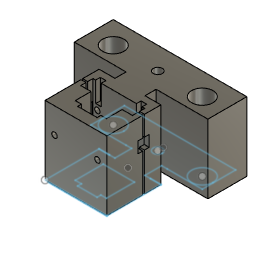
CNC_Assembly (Autodesk Fusion 360 archive; units mm, degrees)
design "spindle handle"
Autodesk Fusion 360 part; units mm, degrees
sketch "Sketch1" plane through (0, 0, 0) normal (0, 0, 1) x (1, 0, 0)
  line L0 (-27.75, -46.75) -> (27.75, -46.75)
  line L1 (27.75, 1.75) -> (27.75, -46.75)
  line L2 (27.75, -46.75) -> (-27.75, -46.75)
  line L3 (14, -8.25) -> (-14, -8.25)
  line L4 (-14, -8.25) -> (-14, -33.35)
  line L5 (-8.5, -36.75) -> (9, -36.75)
  line L6 (14, -33.35) -> (14, -8.25)
  line L7 (-8.5, -36.75) -> (-8.5, -33.35)
  line L8 (-8.5, -33.35) -> (-14, -33.35)
  line L9 (9, -36.75) -> (9, -33.35)
  line L10 (9, -33.35) -> (14, -33.35)
  line L11 (-27.75, 1.75) -> (-18.5, 1.75)
  line L12 (27.75, 1.75) -> (18.5, 1.75)
  circle A0 centre (0, 26.75) radius 4.05
  circle A1 centre (-40, 26.75) radius 9.55
  circle A2 centre (40, 26.75) radius 9.55
  line L13 (50, 46.75) -> (-50, 46.75)
  line L14 (-50, 46.75) -> (-50, 16.75)
  line L15 (50, 16.75) -> (50, 46.75)
  line L16 (-27.75, 1.75) -> (-27.75, -46.75)
  line L17 (-50, 16.75) -> (-18.5, 16.75)
  line L18 (18.5, 16.75) -> (50, 16.75)
  line L19 (-27.75, 1.75) -> (-18.5, 1.75)
  line L20 (18.5, 1.75) -> (27.75, 1.75)
  line L21 (-13.5, 16.75) -> (-13.5, 1.75)
  line L22 (13.5, 1.75) -> (13.5, 16.75)
  line L23 (-18.5, 16.75) -> (-13.5, 16.75)
  line L24 (-18.5, 1.75) -> (-13.5, 1.75)
  line L25 (13.5, 1.75) -> (18.5, 1.75)
  line L26 (13.5, 16.75) -> (18.5, 16.75)
  point P0 (0, 31.75)
  dimension "d19" = 55.5
  dimension "d21" = 48.5
  dimension "d28" = 9.25
  dimension "d29" = 9.25
  dimension "d30" = 15
  dimension "d32" = 8.1
  dimension "d34" = 19.1
  dimension "d36" = 19.1
  dimension "d37" = 100
  dimension "d38" = 30
  dimension "d57" = 27
  dimension "d58" = 15
  dimension "d112" = 28
  dimension "d113" = 17.5
  constraint horizontal L19
  constraint vertical L1
  constraint horizontal L2
  constraint horizontal L3
  constraint perpendicular L3 L4
  constraint parallel L3 L5
  constraint parallel L4 L6
  constraint vertical L7
  constraint horizontal L8
  constraint vertical L9
  constraint horizontal L10
  constraint perpendicular L1 L12
  constraint horizontal L13
  constraint perpendicular L13 L14
  constraint parallel L13 L17
  constraint parallel L14 L15
  constraint collinear L17 L18
  constraint collinear L19 L20
  constraint parallel L21 L22
  constraint perpendicular L21 L23
  measures "d19" distance of L0.start L0.end
  measures "d21" distance of L0.start L11.start
  measures "d28" distance of L11.start L11.end
  measures "d29" distance of L1.start L12.end
  measures "d30" distance of L12.end L18.start
  measures "d32" diameter of A0
  measures "d34" diameter of A1
  measures "d36" diameter of A2
  measures "d37" distance of L14.end L15.start
  measures "d38" distance of L13.end L14.end
  measures "d57" distance of L21.end L22.start
  measures "d58" distance of L21.start L21.end
  measures "d112" distance of L3.start L3.end
  measures "d113" distance of L5.start L5.end
extrude "Extrude4" add sketch "Sketch1" along normal blind 62 makes body 1
sketch "Sketch6" plane through (0, 1.75, 0) normal (0, 1, 0) x (-1, 0, 0)
  line L0 (-27.75, 0) -> (-13.5, 0)
  line L1 (-13.5, 0) -> (-13.5, 62)
  line L2 (-13.5, 62) -> (-27.75, 62)
  line L3 (-27.75, 62) -> (-27.75, 0)
  circle A0 centre (-19.3, 39.2) radius 2.45
  dimension "d63" = 4.9
  measures "d63" diameter of A0
extrude "Extrude5" cut sketch "Sketch6" against normal blind 15 contours A0 bodies 1
sketch "Sketch7" plane through (0, 1.75, 0) normal (0, 1, 0) x (-1, 0, 0)
  line L0 (13.5, 0) -> (27.75, 0)
  line L1 (27.75, 0) -> (27.75, 62)
  line L2 (27.75, 62) -> (13.5, 62)
  line L3 (13.5, 62) -> (13.5, 0)
  circle A0 centre (19.3, 39.2) radius 2.45
  dimension "d71" = 4.9
  measures "d71" diameter of A0
extrude "Extrude6" cut sketch "Sketch7" against normal blind 15 contours A0 bodies 1
sketch "Sketch8" plane through (0, 0, 62) normal (0, 0, 1) x (-1, 0, 0)
  circle A0 centre (0, -26.75) radius 4.05
  circle A1 centre (40, -26.75) radius 9.55
  line L0 (-9, 36.75) -> (8.5, 36.75)
  line L1 (8.5, 36.75) -> (8.5, 33.35)
  line L2 (8.5, 33.35) -> (14, 33.35)
  line L3 (14, 33.35) -> (14, 8.25)
  line L4 (14, 8.25) -> (-14, 8.25)
  line L5 (-14, 8.25) -> (-14, 33.35)
  line L6 (-14, 33.35) -> (-9, 33.35)
  line L7 (-9, 33.35) -> (-9, 36.75)
  circle A2 centre (-40, -26.75) radius 9.55
  line L8 (-13.5, -1.75) -> (-13.5, -16.75)
  line L9 (-13.5, -16.75) -> (-50, -16.75)
  line L10 (-50, -16.75) -> (-50, -46.75)
  line L11 (-50, -46.75) -> (50, -46.75)
  line L12 (50, -46.75) -> (50, -16.75)
  line L13 (50, -16.75) -> (13.5, -16.75)
  line L14 (13.5, -16.75) -> (13.5, -1.75)
  line L15 (13.5, -1.75) -> (27.75, -1.75)
  line L16 (27.75, -1.75) -> (27.75, 46.75)
  line L17 (27.75, 46.75) -> (-27.75, 46.75)
  line L18 (-27.75, 46.75) -> (-27.75, -1.75)
  line L19 (-27.75, -1.75) -> (-13.5, -1.75)
  line L20 (14, 8.25) -> (23.25, 8.25)
  line L21 (23.25, 8.25) -> (23.25, 19.25)
  line L22 (23.25, 19.25) -> (14, 19.25)
  line L23 (14, 19.25) -> (14, 8.25)
  line L24 (-14, 8.25) -> (-23.25, 8.25)
  line L25 (-23.25, 8.25) -> (-23.25, 19.25)
  line L26 (-23.25, 19.25) -> (-14, 19.25)
  line L27 (-14, 19.25) -> (-14, 8.25)
  dimension "d74" = 9.25
  dimension "d75" = 11
  dimension "d76" = 9.25
  dimension "d77" = 11
  constraint horizontal L20
  constraint vertical L21
  constraint horizontal L22
  constraint vertical L23
  constraint coincident L3.end L4.start
  constraint horizontal L24
  constraint vertical L25
  constraint horizontal L26
  constraint vertical L27
  constraint coincident L4.end L5.start
  measures "d74" distance of L3.end L20.end
  measures "d75" distance of L3.end L22.end
  measures "d76" distance of L4.end L24.end
  measures "d77" distance of L4.end L26.end
extrude "Extrude7" cut sketch "Sketch8" against normal blind 35 contours L5 L24 L25 L26 L27 | L3 L20 L21 L22 L23 bodies 1
sketch "Sketch9" plane through (-27.75, 0, 0) normal (-1, 0, 0) x (0, -1, 0)
  line L0 (-1.75, 0) -> (46.75, 0)
  line L1 (46.75, 0) -> (46.75, 62)
  line L2 (46.75, 62) -> (-1.75, 62)
  line L3 (-1.75, 62) -> (-1.75, 0)
sketch "Sketch10" plane through (23.25, 0, 0) normal (-1, 0, 0) x (0, -1, 0)
  line L0 (19.25, 62) -> (8.25, 62)
  line L1 (8.25, 62) -> (8.25, 27)
  line L2 (8.25, 27) -> (19.25, 27)
  line L3 (19.25, 27) -> (19.25, 62)
  line L4 (18.75, 44.2) -> (8.75, 44.2)
  line L5 (8.75, 44.2) -> (8.75, 34.2)
  line L6 (8.75, 34.2) -> (18.75, 34.2)
  line L7 (18.75, 34.2) -> (18.75, 44.2)
  line L8 (18.75, 44.2) -> (8.75, 34.2) construction
  line L9 (8.75, 44.2) -> (18.75, 34.2) construction
  point P0 (13.75, 39.2)
  dimension "d81" = 10
  dimension "d82" = 10
  constraint horizontal L4
  constraint perpendicular L4 L5
  constraint parallel L4 L6
  constraint parallel L5 L7
  constraint coincident L8 P0
  constraint coincident L9 P0
  measures "d81" distance of L5.end L6.end
  measures "d82" distance of L4.end L5.end
extrude "Extrude8" cut sketch "Sketch10" along normal blind 95 and the other way blind 35 contours L4 L5 L6 L7 bodies 1
sketch "Sketch11" plane through (0, 0, 62) normal (0, 0, 1) x (-1, 0, 0)
  line L0 (-23.25, 19.25) -> (-14, 19.25)
  line L1 (-14, 19.25) -> (-14, 33.35)
  line L2 (-14, 33.35) -> (-9, 33.35)
  line L3 (-9, 33.35) -> (-9, 36.75)
  line L4 (-9, 36.75) -> (8.5, 36.75)
  line L5 (8.5, 36.75) -> (8.5, 33.35)
  line L6 (8.5, 33.35) -> (14, 33.35)
  line L7 (14, 33.35) -> (14, 19.25)
  line L8 (14, 19.25) -> (23.25, 19.25)
  line L9 (23.25, 19.25) -> (23.25, 8.25)
  line L10 (23.25, 8.25) -> (-23.25, 8.25)
  line L11 (-23.25, 8.25) -> (-23.25, 19.25)
  circle A0 centre (0, -26.75) radius 4.05
  circle A1 centre (40, -26.75) radius 9.55
  circle A2 centre (-40, -26.75) radius 9.55
  line L12 (-13.5, -1.75) -> (-13.5, -16.75)
  line L13 (-13.5, -16.75) -> (-50, -16.75)
  line L14 (-50, -16.75) -> (-50, -46.75)
  line L15 (-50, -46.75) -> (50, -46.75)
  line L16 (50, -46.75) -> (50, -16.75)
  line L17 (50, -16.75) -> (13.5, -16.75)
  line L18 (13.5, -16.75) -> (13.5, -1.75)
  line L19 (13.5, -1.75) -> (27.75, -1.75)
  line L20 (27.75, -1.75) -> (27.75, 46.75)
  line L21 (27.75, 46.75) -> (-27.75, 46.75)
  line L22 (-27.75, 46.75) -> (-27.75, -1.75)
  line L23 (-27.75, -1.75) -> (-13.5, -1.75)
  line L24 (-33.25, 14.5) -> (-13.25, 14.5)
  line L25 (-13.25, 14.5) -> (-13.25, 13)
  line L26 (-13.25, 13) -> (-33.25, 13)
  line L27 (-33.25, 13) -> (-33.25, 14.5)
  line L28 (-33.25, 14.5) -> (-13.25, 13) construction
  line L29 (-13.25, 14.5) -> (-33.25, 13) construction
  line L30 (13.25, 13) -> (33.25, 13)
  line L31 (33.25, 13) -> (33.25, 14.5)
  line L32 (33.25, 14.5) -> (13.25, 14.5)
  line L33 (13.25, 14.5) -> (13.25, 13)
  line L34 (13.25, 13) -> (33.25, 14.5) construction
  line L35 (33.25, 13) -> (13.25, 14.5) construction
  point P0 (-23.25, 13.75)
  point P1 (23.25, 13.75)
  dimension "d87" = 20
  dimension "d88" = 1.5
  dimension "d91" = 20
  dimension "d92" = 1.5
  constraint horizontal L24
  constraint perpendicular L24 L25
  constraint parallel L24 L26
  constraint parallel L25 L27
  constraint coincident L28 P0
  constraint coincident L29 P0
  constraint midpoint L11 P0
  constraint horizontal L30
  constraint perpendicular L30 L31
  constraint parallel L30 L32
  constraint parallel L31 L33
  constraint coincident L34 P1
  constraint coincident L35 P1
  constraint midpoint L9 P1
  measures "d87" distance of L25.end L26.end
  measures "d88" distance of L24.end L25.end
  measures "d91" distance of L31.end L32.end
  measures "d92" distance of L30.end L31.end
extrude "Extrude9" cut sketch "Sketch11" along normal through all and the other way through all contours L11 L24 L25 L26 | L11 L22 L24 L26 | L22 L24 L26 L27 bodies 1
extrude "Extrude10" cut sketch "Sketch11" along normal through all and the other way through all contours L9 L30 L32 L33 | L9 L20 L30 L32 | L20 L30 L31 L32 bodies 1 makes body 2 at (-9.25, -46.75, 20.6667)
extrude "Extrude11" cut sketch "Sketch6" against normal blind 54 contours A0 bodies 2
extrude "Extrude12" cut sketch "Sketch7" against normal blind 60 contours A0 bodies 2
extrude "Extrude13" add 1 faces at (-50, 36.75, 20.6667) along direction (-1, 0, 0) blind 10 on bodies 1 bodies 1
extrude "Extrude14" add 1 faces at (50, 26.75, 20.6667) along direction (1, 0, 0) blind 10 on bodies 1 bodies 1
extrude "Extrude15" add 1 faces at (44.5, 16.75, 41.3333) along direction (0, -1, 0) blind 5 on bodies 1 bodies 1
extrude "Extrude16" add 1 faces at (-44.5, 16.75, 41.3333) along direction (0, -1, 0) blind 5 on bodies 1 bodies 1
sketch "Sketch12" plane through (0, -8.25, 0) normal (0, -1, 0) x (1, 0, 0)
  circle A0 centre (19.3, 39.2) radius 2.45
  circle A1 centre (-19.3, 39.2) radius 2.45
  line L0 (-14, 0) -> (14, 0)
  line L1 (14, 0) -> (14, 27)
  line L2 (14, 27) -> (23.25, 27)
  line L3 (23.25, 27) -> (23.25, 62)
  line L4 (23.25, 62) -> (-23.25, 62)
  line L5 (-23.25, 62) -> (-23.25, 27)
  line L6 (-23.25, 27) -> (-14, 27)
  line L7 (-14, 27) -> (-14, 0)
  line L8 (20.8, 64.3767) -> (15.8178, 64.3767)
  line L9 (-15.8178, 65.2934) -> (-20.8, 65.2934)
  line L10 (-15.8178, 43.7) -> (-20.8, 43.7)
  line L11 (20.8, 43.7) -> (15.8178, 43.7)
  line L12 (20.8, 43.7) -> (20.8, 64.3767)
  line L13 (15.8178, 64.3767) -> (15.8178, 43.7)
  line L14 (-15.8178, 43.7) -> (-15.8178, 65.2934)
  line L15 (-20.8, 65.2934) -> (-20.8, 43.7)
  point P0 (19.3, 39.2)
  point P1 (-19.3, 39.2)
  constraint horizontal L8
  constraint perpendicular L8 L13
  constraint coincident P0 A0.centre
  constraint horizontal L9
  constraint perpendicular L9 L15
  constraint coincident P1 A1.centre
extrude "Extrude17" cut sketch "Sketch12" against normal blind 4.2 contours L4 L9 L14 L15 | L4 L10 L14 L15 | L4 L11 L12 L13 | L4 L8 L12 L13 bodies 1
sketch "Sketch2" plane through (0, 0, 60) normal (0, 0, 1) x (-1, 0, 0)
  circle A0 centre (0, -26.75) radius 4
  circle A1 centre (-40, -26.75) radius 5
  line L0 (-8.5, 36.75) -> (8.5, 36.75)
  line L1 (8.5, 36.75) -> (8.5, 33.35)
  line L2 (8.5, 33.35) -> (13.5, 33.35)
  line L3 (13.5, 33.35) -> (13.5, 8.25)
  line L4 (13.5, 8.25) -> (-13.5, 8.25)
  line L5 (-13.5, 8.25) -> (-13.5, 33.35)
  line L6 (-13.5, 33.35) -> (-8.5, 33.35)
  line L7 (-8.5, 33.35) -> (-8.5, 36.75)
  circle A2 centre (40, -26.75) radius 5
  line L8 (-18.5, -16.75) -> (-50, -16.75)
  line L9 (-50, -16.75) -> (-50, -46.75)
  line L10 (-50, -46.75) -> (50, -46.75)
  line L11 (50, -46.75) -> (50, -16.75)
  line L12 (50, -16.75) -> (18.5, -16.75)
  line L13 (18.5, -16.75) -> (18.5, -1.75)
  line L14 (18.5, -1.75) -> (27.75, -1.75)
  line L15 (27.75, -1.75) -> (27.75, 46.75)
  line L16 (27.75, 46.75) -> (-27.75, 46.75)
  line L17 (-27.75, 46.75) -> (-27.75, -1.75)
  line L18 (-27.75, -1.75) -> (-18.5, -1.75)
  line L19 (-18.5, -1.75) -> (-18.5, -16.75)
  line L20 (-13.5, 8.25) -> (-22.79, 8.25)
  line L21 (-22.79, 8.25) -> (-22.79, 19.25)
  line L22 (-22.79, 19.25) -> (-13.5, 19.25)
  line L23 (-13.5, 19.25) -> (-13.5, 8.25)
  line L24 (13.5, 8.25) -> (22.75, 8.25)
  line L25 (22.75, 8.25) -> (22.75, 19.25)
  line L26 (22.75, 19.25) -> (13.5, 19.25)
  line L27 (13.5, 19.25) -> (13.5, 8.25)
  dimension "d41" = 9.29
  dimension "d42" = 11
  dimension "d43" = 9.25
  dimension "d44" = 11
  constraint horizontal L20
  constraint vertical L21
  constraint horizontal L22
  constraint vertical L23
  constraint coincident L4.end L5.start
  constraint horizontal L24
  constraint vertical L25
  constraint horizontal L26
  constraint vertical L27
  constraint coincident L3.end L4.start
  measures "d41" distance of L4.end L20.end
  measures "d42" distance of L4.end L22.end
  measures "d43" distance of L3.end L24.end
  measures "d44" distance of L3.end L26.end
sketch "Sketch3" plane through (0, 0, 0) normal (0, 1, 0) x (1, 0, 0)

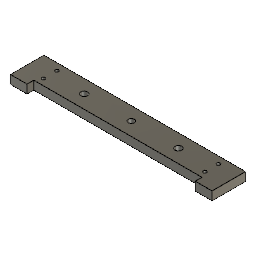
design "X Axis"
Autodesk Fusion 360 part; units mm, degrees
sketch "Sketch1" plane through (0, 0, 0) normal (0, 0, 1) x (1, 0, 0)
  line L0 (150, -20) -> (-150, -20)
  line L1 (-150, -20) -> (-150, 20)
  line L2 (-150, 20) -> (150, 20)
  line L3 (150, 20) -> (150, -20)
  line L4 (150, -20) -> (-150, 20) construction
  line L5 (-150, -20) -> (150, 20) construction
  dimension "d4" = 40
  dimension "d5" = 300
  constraint horizontal L0
  constraint perpendicular L0 L1
  constraint parallel L0 L2
  constraint parallel L1 L3
  constraint coincident L4 origin
  constraint coincident L5 origin
  measures "d4" distance of L0.end L1.end
  measures "d5" distance of L0.start L0.end
extrude "Extrude1" add sketch "Sketch1" along normal blind 13
sketch "Sketch2" plane through (0, 0, 0) normal (0, 0, 1) x (1, 0, 0)
  circle A0 centre (0, 0) radius 4.5
  circle A1 centre (-70, 0) radius 5
  circle A2 centre (70, 0) radius 5
  circle A3 centre (-120, 9.4) radius 2.5
  circle A4 centre (-120, -10.6) radius 2.5
  line L0 (-120, 9.4) -> (-120, 19.8) construction
  line L1 (-120, -10.6) -> (-120, -21) construction
  line L2 (0, -20) -> (0, 20) construction
  circle A5 centre (120, 9.4) radius 2.5
  circle A6 centre (120, -10.6) radius 2.5
  line L3 (-150, 20) -> (-150, -20)
  dimension "d8" = 9
  dimension "d9" = 10
  dimension "d10" = 10
  dimension "d11" = 70
  dimension "d12" = 70
  dimension "d13" = 5
  dimension "d14" = 5
  dimension "d15" = 20
  dimension "d22" = 30
  constraint coincident A0.centre origin
  constraint coincident A3.centre L0.start
  constraint vertical L0
  constraint coincident A4.centre L1.start
  constraint vertical L1
  constraint equal L0 L1
  constraint vertical L2
  constraint symmetric A3 L2 A5
  constraint symmetric A4 L2 A6
  constraint coincident A0.centre L2
  measures "d8" diameter of A0
  measures "d9" diameter of A1
  measures "d10" diameter of A2
  measures "d11" distance of A0.centre A1.centre
  measures "d12" distance of A0.centre A2.centre
  measures "d13" diameter of A3
  measures "d14" diameter of A4
  measures "d15" distance of A3.centre A4.centre
  measures "d22" distance of A3.centre L3
extrude "Extrude2" cut sketch "Sketch2" along normal blind 13
sketch "Sketch3" plane through (0, 0, 13) normal (0, 0, 1) x (-1, 0, 0)
  circle A0 centre (70, 0) radius 5
  circle A1 centre (0, 0) radius 4.5
  circle A2 centre (-120, 10.6) radius 2.5
  circle A3 centre (120, -9.4) radius 2.5
  circle A4 centre (-70, 0) radius 5
  circle A5 centre (-120, -9.4) radius 2.5
  circle A6 centre (120, 10.6) radius 2.5
  line L0 (-150, -20) -> (150, -20)
  line L1 (150, -20) -> (150, 20)
  line L2 (150, 20) -> (-150, 20)
  line L3 (-150, 20) -> (-150, -20)
sketch "Sketch5" plane through (0, 0, 13) normal (0, 0, 1) x (-1, 0, 0)
  line L0 (150, 20) -> (125, 20)
  line L1 (125, 20) -> (125, 30)
  line L2 (125, 30) -> (150, 30)
  line L3 (150, 30) -> (150, 20)
  line L4 (-150, -20) -> (150, -20)
  line L5 (0, -20) -> (0, 50) construction
  line L6 (-150, 20) -> (-125, 20)
  line L7 (-150, 30) -> (-150, 20)
  line L8 (-125, 30) -> (-150, 30)
  line L9 (-125, 20) -> (-125, 30)
  point P0 (150, 20)
  dimension "d23" = 10
  dimension "d24" = 25
  constraint horizontal L0
  constraint vertical L1
  constraint horizontal L2
  constraint vertical L3
  constraint coincident P0 L0.start
  constraint midpoint L4 L5.start
  constraint perpendicular L4 L5
  constraint symmetric P0 L5 L6.start
  constraint symmetric L0.end L5 L6.end
  constraint symmetric L1.end L5 L8.start
  constraint symmetric L2.end L5 L7.start
  measures "d23" distance of L0.end L1.end
  measures "d24" distance of L1.end L2.end
extrude "Extrude4" add sketch "Sketch5" against normal blind 13
sketch "Sketch4" plane through (0, 0, 13) normal (0, 0, 1) x (-1, 0, 0)
  line L0 (150, 20) -> (125, 20)
  line L1 (125, 20) -> (125, 30)
  line L2 (125, 30) -> (150, 30)
  line L3 (150, 30) -> (150, 20)
  line L4 (-150, -20) -> (150, -20)
  line L5 (0, -20) -> (0, 50) construction
  line L6 (-150, 20) -> (-125, 20)
  line L7 (-150, 30) -> (-150, 20)
  line L8 (-125, 30) -> (-150, 30)
  line L9 (-125, 20) -> (-125, 30)
  point P0 (150, 20)
  dimension "d18" = 10
  dimension "d19" = 25
  constraint horizontal L0
  constraint vertical L1
  constraint horizontal L2
  constraint vertical L3
  constraint coincident P0 L0.start
  constraint midpoint L4 L5.start
  constraint symmetric P0 L5 L6.start
  constraint symmetric L0.end L5 L6.end
  constraint symmetric L1.end L5 L8.start
  constraint symmetric L2.end L5 L7.start
  measures "d18" distance of L0.end L1.end
  measures "d19" distance of L1.end L2.end
extrude "Extrude3" [suppressed]
equation "thickness = 13 mm"
equation "lenght = 300 mm"
equation "width = 40 mm"
equation "d4 = width"
equation "d5 = lenght"
equation "d6 = thickness"
equation "d16 = thickness"

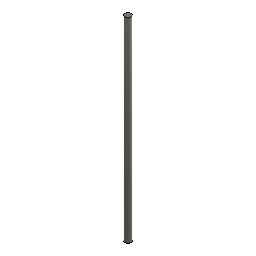
design "10mm rod 300mm"
Autodesk Fusion 360 part; units mm, degrees
sketch "Sketch1" plane through (0, 0, 0) normal (0, 1, 0) x (1, 0, 0)
  circle A0 centre (0, 0) radius 5
  dimension "d3" = 10
  constraint coincident A0.centre origin
  measures "d3" diameter of A0
extrude "Extrude1" add sketch "Sketch1" along normal blind 300
equation "D = 10 mm"
equation "Lenght = 300 mm"
equation "d3 = D"
equation "d4 = Lenght"

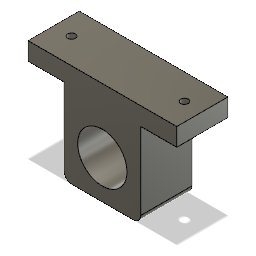
design "X Axis Rail Support"
Autodesk Fusion 360 part; units mm, degrees
sketch "Sketch1" plane through (0, 0, 0) normal (0, 0, 1) x (1, 0, 0)
  line L0 (-4, 26.4315) -> (26, 26.4315)
  line L1 (26, 26.4315) -> (26, -13.5685)
  line L2 (26, -13.5685) -> (-4, -13.5685)
  line L3 (-4, -13.5685) -> (-4, 26.4315)
  line L4 (-4, 26.4315) -> (-18, 26.4315)
  line L5 (-18, 26.4315) -> (-18, 19.4315)
  line L6 (-18, 19.4315) -> (-4, 19.4315)
  line L7 (-4, 19.4315) -> (-4, 26.4315)
  circle A0 centre (11, 6.4315) radius 9.6
  line L8 (11, 26.4315) -> (11, -13.5685)
  line L9 (26, 6.4315) -> (-4, 6.4315)
  line L10 (26, 26.4315) -> (40, 26.4315)
  line L11 (26, 19.4315) -> (26, 26.4315)
  line L12 (40, 26.4315) -> (40, 19.4315)
  line L13 (40, 19.4315) -> (26, 19.4315)
  dimension "d7" = 30
  dimension "d8" = 40
  dimension "d9" = 14
  dimension "d10" = 7
  dimension "d23" = 19.2
  constraint horizontal L0
  constraint vertical L1
  constraint horizontal L2
  constraint vertical L3
  constraint horizontal L4
  constraint vertical L5
  constraint horizontal L6
  constraint vertical L7
  constraint midpoint L0 L8.start
  constraint midpoint L2 L8.end
  constraint midpoint L1 L9.start
  constraint midpoint L3 L9.end
  constraint symmetric L0.start L8 L0.end
  constraint symmetric L4.end L8 L10.end
  constraint symmetric L5.end L8 L12.end
  constraint symmetric L6.end L8 L11.start
  constraint coincident A0.centre L8
  constraint coincident A0.centre L9
  measures "d7" distance of L1 L3
  measures "d8" distance of L0 L2
  measures "d9" distance of L5 L7
  measures "d10" distance of L4 L6
  measures "d23" diameter of A0
ref_plane "WorkPlane1" through (33, 16.9315, 10) normal (0, -1, 0) x (1, 0, 0)
sketch "Sketch3" plane through (33, 16.9315, 10) normal (0, -1, 0) x (1, 0, 0)
  line L0 (0, 10) -> (0, -10)
  line L1 (7, 0) -> (-7, 0)
  circle A0 centre (0, 0) radius 1.5
  line L2 (-44, 10) -> (-44, -10)
  line L3 (-51, 0) -> (-37, 0)
  circle A1 centre (-44, 0) radius 1.5
  dimension "d33" = 3
  dimension "d34" = 3
  constraint vertical L0
  constraint perpendicular L0 L1
  constraint coincident A0.centre origin
  constraint vertical L2
  constraint horizontal L3
  constraint midpoint L3 A1.centre
  measures "d33" diameter of A0
  measures "d34" diameter of A1
extrude "Extrude6" add sketch "Sketch1" along normal blind 20 contours L0 L3 L7 A0 L8 L9 | L3 L4 L5 L6 L7 | L0 L1 A0 L8 L9 L11 | L1 L10 L11 L12 L13 | L2 L3 A0 L8 L9 | L1 L2 A0 L8 L9
extrude "Extrude7" cut sketch "Sketch3" along normal mid plane 40
fillet "Fillet7" radius 3 1 edges at (26, -13.5685, 10)
fillet "Fillet8" radius 3 1 edges at (-4, -13.5685, 10)
move_face "MoveFace2" to x (1, 0, 0) y (0, 1, 0) z (0, 0, 1) at (0, -5, 0) 1 faces at (20.5523, 5.4756, 6.6667)
equation "R1 = 19.20 mm"
equation "R2 = 3 mm"
equation "height = 40 mm"
equation "lenght = 20 mm"
equation "width = 30 mm"
equation "width2 = 7 mm"
equation "d7 = width"
equation "d8 = height"
equation "d9 = width2 * 2"
equation "d10 = width2"
equation "d23 = R1"
equation "d33 = R2"
equation "d34 = R2"
equation "d41 = lenght"
equation "d43 = lenght"
equation "d46 = R2"
equation "d48 = R2"

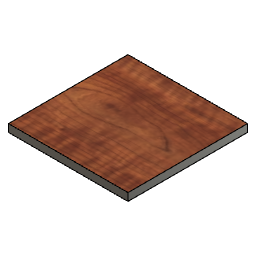
design "x axis bed"
Autodesk Fusion 360 part; units mm, degrees
sketch "Sketch1" plane through (0, 0, 0) normal (0, 1, 0) x (1, 0, 0)
  line L0 (-200, 50) -> (50, 50)
  line L1 (50, 50) -> (50, -200)
  line L2 (50, -200) -> (-200, -200)
  line L3 (-200, -200) -> (-200, 50)
  dimension "d4" = 250
  dimension "d5" = 250
  constraint horizontal L0
  constraint vertical L1
  constraint horizontal L2
  constraint vertical L3
  measures "d4" distance of L0 L2
  measures "d5" distance of L1 L3
extrude "Extrude1" add sketch "Sketch1" along normal blind 16
move_face "MoveFace1" by (0, 0, -130) 1 faces at (-116.6667, 16, 33.3333)
equation "th = 16 mm"
equation "lenght = 250 mm"
equation "width = 250 mm"
equation "d4 = lenght"
equation "d5 = width"
equation "d6 = th"

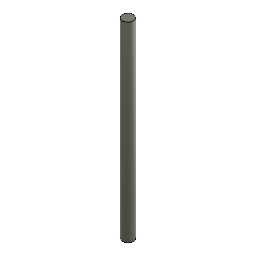
design "10mm rod 170mm"
Autodesk Fusion 360 part; units mm, degrees
sketch "Sketch1" plane through (0, 0, 0) normal (0, 1, 0) x (1, 0, 0)
  circle A0 centre (0, 0) radius 5
  dimension "d3" = 10
  constraint coincident A0.centre origin
  measures "d3" diameter of A0
extrude "Extrude1" add sketch "Sketch1" along normal blind 170
equation "D = 10 mm"
equation "Lenght = 170 mm"
equation "d3 = D"
equation "d4 = Lenght"

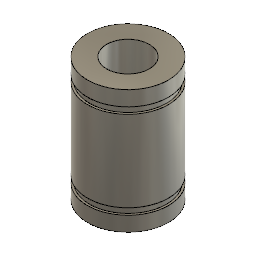
design "10mm Linear Ball Bearing"
Autodesk Fusion 360 part; units mm, degrees
sketch "Sketch1" plane through (0, 0, 0) normal (0, 1, 0) x (1, 0, 0)
  circle A0 centre (0, 0) radius 5
  circle A1 centre (0, 0) radius 9.5
  dimension "d4" = 10
  dimension "d5" = 19
  constraint coincident A0.centre A1.centre
  constraint concentric A0 A1
  measures "d4" diameter of A0
  measures "d5" diameter of A1
extrude "Extrude1" add sketch "Sketch1" along normal blind 29 makes body 1
sketch "Sketch2" plane through (0, 0, 0) normal (0, 0, 1) x (1, 0, 0)
  line L0 (9.5, 3.5) -> (9, 3.5)
  line L1 (9, 3.5) -> (9, 5)
  line L2 (9, 5) -> (9.5, 5)
  line L3 (9.5, 5) -> (9.5, 3.5)
  line L4 (9.5, 25.5) -> (9, 25.5)
  line L5 (9, 25.5) -> (9, 24)
  line L6 (9, 24) -> (9.5, 24)
  line L7 (9.5, 24) -> (9.5, 25.5)
  line L8 (9.5, 0) -> (-9.5, 0)
  line L9 (9.5, 29) -> (-9.5, 29)
  dimension "d8" = 3.5
  dimension "d9" = 3.5
  dimension "d10" = 1.5
  dimension "d11" = 0.5
  dimension "d12" = 1.5
  dimension "d13" = 0.5
  constraint horizontal L0
  constraint vertical L1
  constraint horizontal L2
  constraint vertical L3
  constraint horizontal L4
  constraint vertical L5
  constraint horizontal L6
  constraint vertical L7
  measures "d8" distance of L0.start L8
  measures "d9" distance of L4.start L9
  measures "d10" distance of L4.start L6.end
  measures "d11" distance of L4.start L4.end
  measures "d12" distance of L0.start L2.end
  measures "d13" distance of L0.start L0.end
revolve "Revolve1" cut sketch "Sketch2" angle 360 about axis through (0, 0, 0) along (0, -1, 0) bodies 1
copy_body "Body->Comp1" bodies 1 removing the originals makes body 2 in component "Component"
component "Component" placed x (1, 0, 0) y (0, 1, 0) z (0, 0, 1) at (0, 0, 0)
equation "InnerD = 10 mm"
equation "OuterDiameter = 19 mm"
equation "Lenght = 29 mm"
equation "d4 = InnerD"
equation "d5 = OuterDiameter"
equation "d6 = Lenght"

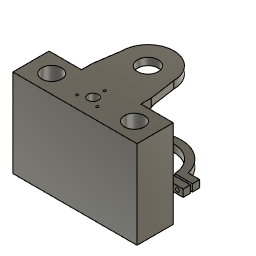
design "SPINDLE HANDLE FOR DREMEL"
Autodesk Fusion 360 part; units mm, degrees
sketch "Sketch1" plane through (0, 0, 0) normal (0, 0, 1) x (1, 0, 0)
  line L0 (60, 17.5) -> (-60, 17.5)
  line L1 (-60, 17.5) -> (-60, -17.5)
  line L2 (-60, -17.5) -> (60, -17.5)
  line L3 (60, -17.5) -> (60, 17.5)
  line L4 (60, 17.5) -> (-60, -17.5) construction
  line L5 (-60, 17.5) -> (60, -17.5) construction
  line L6 (28.75, 27.5) -> (-28.75, 7.5) construction
  line L7 (-28.75, 27.5) -> (28.75, 7.5) construction
  line L8 (28.75, 7.5) -> (28.75, 8.3854)
  line L9 (28.75, 17.5) -> (28.75, 27.5)
  line L10 (-28.75, 27.5) -> (-28.75, 17.5)
  line L11 (-28.75, 8.3854) -> (-28.75, 7.5)
  line L12 (-31.242, 60.75) -> (-42.25, 60.75)
  line L13 (-42.25, 44.75) -> (-31.242, 44.75)
  line L14 (-24.4711, 58.9731) -> (-33.5, 51.75) construction
  line L15 (-42.25, 60.75) -> (-24.4711, 46.5269) construction
  line L16 (42.25, 60.75) -> (31.242, 60.75)
  line L17 (42.25, 53.75) -> (25.2302, 53.75)
  line L18 (-25.2302, 53.75) -> (-42.25, 53.75)
  line L19 (-42.25, 51.75) -> (-25.2302, 51.75)
  line L20 (-25.2403, 53.451) -> (-32.25, 52.75) construction
  line L21 (-32.25, 52.75) -> (-25.2403, 52.049) construction
  line L22 (42.25, 60.75) -> (33.5, 53.75) construction
  line L23 (31, 51.75) -> (22.25, 44.75) construction
  line L24 (24.4711, 58.9731) -> (31, 53.75) construction
  line L25 (33.5, 51.75) -> (42.25, 44.75) construction
  line L26 (25.2302, 51.75) -> (31, 51.75)
  line L27 (33.5, 51.75) -> (42.25, 51.75)
  line L28 (42.25, 44.75) -> (42.25, 51.75)
  line L29 (42.25, 53.75) -> (42.25, 60.75)
  line L30 (33.5, 51.75) -> (31, 51.75)
  line L31 (22.25, 44.75) -> (23.9492, 44.75)
  line L32 (31.242, 44.75) -> (42.25, 44.75)
  arc A0 (25.2302, 53.75) -> (-25.2302, 53.75) centre (0, 52.75) ccw
  arc A1 (-25.2302, 51.75) -> (25.2302, 51.75) centre (0, 52.75) ccw
  arc A2 (31.242, 60.75) -> (-31.242, 60.75) centre (0, 52.75) ccw
  line L33 (-42.25, 60.75) -> (-42.25, 53.75)
  line L34 (-42.25, 51.75) -> (-42.25, 44.75)
  arc A3 (-31.242, 44.75) -> (-20.0624, 27.5) centre (0, 52.75) ccw
  arc A4 (20.0624, 27.5) -> (31.242, 44.75) centre (0, 52.75) ccw
  line L35 (28.75, 27.5) -> (20.0624, 27.5)
  line L36 (-20.0624, 27.5) -> (-28.75, 27.5)
  circle A5 centre (0, 0) radius 5
  circle A6 centre (-40, 0) radius 9.55
  circle A7 centre (40, 0) radius 9.55
  circle A8 centre (9.7967, -5.6561) radius 2.125
  circle A9 centre (0, 11.3123) radius 2.125
  line L37 (-12.8278, -7.4061) -> (-9.7967, -5.6561) construction
  line L38 (0, 0) -> (8.4764, 4.8939) construction
  line L39 (0, 14.8123) -> (0, 11.3123) construction
  line L40 (12.8278, -7.4061) -> (9.7967, -5.6561) construction
  line L41 (0, 0) -> (-8.4764, 4.8939) construction
  circle A10 centre (-9.7967, -5.6561) radius 2.125
  line L42 (0, 0) -> (0, -9.7877) construction
  circle A11 centre (0, 11.3123) radius 1.125
  circle A12 centre (9.7967, -5.6561) radius 1.125
  circle A13 centre (-9.7967, -5.6561) radius 1.125
  point P0 (0, 17.5)
  point P1 (-32.25, 52.75)
  point P2 (32.25, 52.75)
  point P3 (32.25, 52.75)
  point P4 (-32.25, 52.75)
  dimension "d1" = 120
  dimension "d2" = 35
  dimension "d3" = 57.5
  dimension "d4" = 20
  dimension "d6" = 50.5
  dimension "d9" = 16
  dimension "d10" = 20
  dimension "d13" = 2
  dimension "d14" = 10
  dimension "d15" = 40
  dimension "d16" = 19.1
  dimension "d17" = 40
  dimension "d21" = 4.25
  dimension "d22" = 3.5
  dimension "d30" = -1
  dimension "d31" = -1
  dimension "d32" = -1
  constraint horizontal L0
  constraint perpendicular L0 L1
  constraint parallel L0 L2
  constraint parallel L1 L3
  constraint coincident L4 A5.centre
  constraint coincident L5 A5.centre
  constraint coincident A5.centre L38.start
  constraint horizontal L35
  constraint perpendicular L10 L35
  constraint parallel L8 L10
  constraint coincident L6 P0
  constraint coincident L7 P0
  constraint midpoint L0 P0
  constraint coincident L4 L8.end
  constraint coincident L0 L9.start
  constraint collinear L8 L9
  constraint coincident L0 L10.end
  constraint coincident L5 L11.start
  constraint collinear L10 L11
  constraint coincident P4 A2
  constraint horizontal L12
  constraint perpendicular L12 L33
  constraint parallel L12 L13
  constraint coincident L14 P4
  constraint coincident L15 P4
  constraint coincident P4 P1
  constraint horizontal L16
  constraint parallel L16 L31
  constraint coincident P3 L22
  constraint coincident P3 L24
  constraint horizontal L17
  constraint parallel L17 L26
  constraint coincident P3 P2
  constraint horizontal L18
  constraint parallel L18 L19
  constraint coincident L20 P4
  constraint coincident L21 P4
  constraint collinear L22 L23
  constraint coincident L17 L24.end
  constraint collinear L24 L25
  constraint coincident L25.start L26
  constraint coincident L17 L22.end
  constraint collinear L26 L27
  constraint collinear L28 L29
  constraint coincident L32.start L31
  constraint coincident L24.start A0
  constraint coincident L31.end A0
  constraint collinear L31 L32
  constraint coincident L14.start A0
  constraint coincident L19.end A0
  constraint coincident L21.end A0
  constraint coincident L15.end A0
  constraint coincident L19 L14.end
  constraint concentric A0 A1
  constraint concentric A2 A3
  constraint collinear L33 L34
  constraint coincident A3.end L35
  constraint concentric A3 A4
  constraint collinear L35 L36
  constraint equal A8 A9
  constraint equal A8 A10
  constraint coincident A8.centre L40.end
  constraint coincident L37.end A10.centre
  constraint coincident A9.centre L39.end
  constraint equal L37 L40
  constraint equal L39 L40
  measures "d1" distance of L1.end L2.end
  measures "d2" distance of L0.end L1.end
  measures "d3" distance of L6.end L7.end
  measures "d4" distance of L7.start L6.end
  measures "d6" diameter of A0
  measures "d9" distance of L12.end L13.start
  measures "d10" distance of L23.end L25.end
  measures "d13" distance of L18.end L19.start
  measures "d14" diameter of A5
  measures "d15" distance of A5.centre A6.centre
  measures "d16" diameter of A6
  measures "d17" distance of A5.centre A7.centre
  measures "d21" diameter of A8
  measures "d22" distance of A9.centre L39.start
extrude "Extrude1" add sketch "Sketch1" along normal blind 85 contours L0 L1 L2 L3 | A8 | A9 | A10 | A11 | A12 | A13 makes body 1
extrude "Extrude2" add sketch "Sketch1" along normal blind 7 contours L0 L9 L10 L13 L19 L26 L27 L28 L30 L32 A1 L34 A3 A4 L35 L36 | L12 L16 L17 L18 L29 A0 A2 L33 bodies 1 makes body 2 at (32.9074, 56.0833, 0)
fillet "Fillet1" radius 10 1 edges at (0, 17.5, 7) on bodies 1
extrude "Extrude3" cut sketch "Sketch1" along normal through all contours A11 | A12 | A13 bodies 1
sketch "Sketch2" plane through (0, 0, 85) normal (0, 0, 1) x (-1, 0, 0)
  circle A0 centre (9.7967, 5.6561) radius 1.125
  circle A1 centre (-9.7967, 5.6561) radius 1.125
  circle A2 centre (0, -11.3123) radius 1.125
  circle A3 centre (40, 0) radius 9.55
  circle A4 centre (0, 0) radius 5
  circle A5 centre (-40, 0) radius 9.55
  line L0 (-60, 17.5) -> (-60, -17.5)
  line L1 (-60, -17.5) -> (60, -17.5)
  line L2 (60, -17.5) -> (60, 17.5)
  line L3 (60, 17.5) -> (-60, 17.5)
  line L4 (28.7494, -27.5) -> (28.7494, -17.5)
  line L5 (28.7494, -17.5) -> (-28.75, -17.5)
  line L6 (-28.75, -17.5) -> (-28.75, -27.5)
  circle A6 centre (0, -53) radius 10
  line L7 (-28.75, -27.5) -> (-25, -53)
  line L8 (25, -53) -> (28.7494, -27.5)
  arc A7 (-25, -53) -> (25, -53) centre (0, -53) ccw
  dimension "d34" = 20
  constraint vertical L4
  constraint horizontal L5
  constraint vertical L6
  constraint coincident L1 L4.end
  constraint concentric A6 A7
  measures "d34" diameter of A6
extrude "Extrude4" add sketch "Sketch2" against normal blind 7 contours L1 L4 L5 L6 L7 L8 A7 bodies 1
fillet "Fillet2" radius 15 1 edges at (0.0003, 17.5, 78) on bodies 1
sketch "Sketch3" plane through (0, 60.75, 0) normal (0, 1, 0) x (-1, 0, 0)
  line L0 (-42.25, 0) -> (-31.242, 0)
  line L1 (-31.242, 0) -> (-31.242, 7)
  line L2 (-31.242, 7) -> (-42.25, 7)
  line L3 (-42.25, 7) -> (-42.25, 0)
  circle A0 centre (-36.746, 3.5) radius 1.8
  circle A1 centre (36.5, 3.5) radius 1.8
  dimension "d40" = 3.6
  dimension "d43" = 3.6
  measures "d40" diameter of A0
  measures "d43" diameter of A1
extrude "Extrude5" cut sketch "Sketch3" against normal blind 35 contours A0 | A1 bodies 1 2
